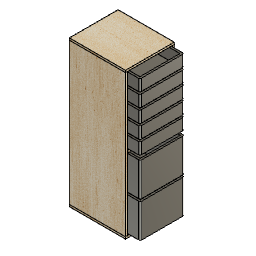
model (Autodesk Fusion 360 design; units mm, degrees)
Autodesk Fusion 360 part; units mm, degrees
note: some values were not read from the file. Chosen so that the rebuilt part matches the saved one: which bodies a step acts on.
sketch "Sketch1" plane through (0, 0, 0) normal (0, 0, 1) x (1, 0, 0) in component "eb432"
  line L0 (15, 0) -> (383, 0)
  line L1 (398, 15) -> (398, 284)
  line L2 (383, 299) -> (15, 299)
  line L3 (0, 284) -> (0, 15)
  arc A0 (15, 299) -> (0, 284) centre (15, 284) ccw
  arc A1 (398, 284) -> (383, 299) centre (383, 284) ccw
  arc A2 (383, 0) -> (398, 15) centre (383, 15) ccw
  arc A3 (0, 15) -> (15, 0) centre (15, 15) ccw
  line L4 (0, 0) -> (18, 18) construction
  line L5 (18, 18) -> (380, 18)
  line L6 (380, 18) -> (380, 281)
  line L7 (380, 281) -> (18, 281)
  line L8 (18, 281) -> (18, 18)
  point P0 (398, 0)
  point P1 (0, 299)
  dimension "d1" = 398
  dimension "d2" = 299
  dimension "d3" = 15
  dimension "d6" = 18
  dimension "d7" = 18
  dimension "d8" = 263
  dimension "d15" = 362
  constraint horizontal L0
  constraint vertical L1
  constraint horizontal L2
  constraint vertical L3
  constraint coincident L4.start origin
  constraint coincident P1 L2
  constraint coincident P1 L3
  constraint tangent L2 A0
  constraint tangent L3 A0
  constraint tangent L1 A1
  constraint tangent L2 A1
  constraint equal A0 A1
  constraint coincident P0 L0
  constraint coincident P0 L1
  constraint tangent L0 A2
  constraint tangent L1 A2
  constraint equal A0 A2
  constraint coincident L4.start L0
  constraint coincident L4.start L3
  constraint tangent L0 A3
  constraint tangent L3 A3
  constraint equal A0 A3
  constraint horizontal L5
  constraint vertical L6
  constraint horizontal L7
  constraint vertical L8
  measures "d1" distance of L4.start P0
  measures "d2" distance of L4.start P1
  measures "d3" radius of A0
  measures "d6" horizontal distance of L4.end L4.start
  measures "d7" vertical distance of L4.end L4.start
  measures "d8" distance of L5.end L6.end
  measures "d15" distance of L6.end L7.end
extrude "Extrude1" add sketch "Sketch1" along normal blind 14 and the other way blind -218 makes body 1 in component "eb432"
extrude "Extrude2" add sketch "Sketch1" along normal blind 14 separate body contours L5 L6 L7 L8 makes body 2 in component "eb432"
sketch "Sketch1 (2)" plane through (0, 0, 0) normal (0, 0, 1) x (1, 0, 0) in component "eb641"
  arc A0 (599, 384) -> (584, 399) centre (584, 384) ccw
  line L0 (0, 384) -> (0, 15)
  line L1 (599, 15) -> (599, 384)
  line L2 (584, 399) -> (15, 399)
  arc A1 (15, 399) -> (0, 384) centre (15, 384) ccw
  arc A2 (0, 15) -> (15, 0) centre (15, 15) ccw
  arc A3 (584, 0) -> (599, 15) centre (584, 15) ccw
  line L3 (581, 381) -> (18, 381)
  line L4 (581, 18) -> (581, 381)
  line L5 (18, 381) -> (18, 18)
  line L6 (18, 18) -> (581, 18)
  line L7 (0, 0) -> (18, 18) construction
  line L8 (15, 0) -> (584, 0)
  point P0 (0, 399)
  point P1 (599, 0)
  dimension "d28" = 599
  dimension "d29" = 399
  dimension "d30" = 15
  dimension "d31" = 18
  dimension "d32" = 18
  dimension "d33" = 363
  dimension "d34" = 563
  constraint horizontal L8
  constraint vertical L1
  constraint horizontal L2
  constraint vertical L0
  constraint coincident L7.start origin
  constraint coincident P0 L2
  constraint coincident P0 L0
  constraint tangent L2 A1
  constraint tangent L0 A1
  constraint tangent A0 L1
  constraint tangent A0 L2
  constraint equal A0 A1
  constraint coincident P1 L8
  constraint coincident P1 L1
  constraint tangent A3 L8
  constraint tangent L1 A3
  constraint equal A1 A3
  constraint coincident L7.start L8
  constraint coincident L7.start L0
  constraint tangent A2 L8
  constraint tangent L0 A2
  constraint equal A1 A2
  constraint horizontal L6
  constraint vertical L4
  constraint horizontal L3
  constraint vertical L5
  measures "d28" distance of P1 L7.start
  measures "d29" distance of P0 L7.start
  measures "d30" radius of A1
  measures "d31" horizontal distance of L7.start L5.end
  measures "d32" vertical distance of L7.start L5.end
  measures "d33" distance of L4.start L3.start
  measures "d34" distance of L3.start L3.end
extrude "Extrude1'" add sketch "Sketch1 (2)" along normal blind 14 separate body contours L3 L4 L5 L6 makes body 3 in component "eb641"
extrude "Extrude2'" add sketch "Sketch1 (2)" along normal blind 14 and the other way blind -118 bodies 3 in component "eb641"
sketch "Sketch1 (3)" plane through (0, 0, 0) normal (0, 0, 1) x (1, 0, 0) in component "eb643"
  line L0 (584, 399) -> (15, 399)
  line L1 (599, 15) -> (599, 384)
  arc A0 (0, 15) -> (15, 0) centre (15, 15) ccw
  line L2 (581, 18) -> (581, 381)
  line L3 (0, 0) -> (18, 18) construction
  line L4 (18, 18) -> (581, 18)
  arc A1 (584, 0) -> (599, 15) centre (584, 15) ccw
  line L5 (15, 0) -> (584, 0)
  arc A2 (599, 384) -> (584, 399) centre (584, 384) ccw
  line L6 (581, 381) -> (18, 381)
  arc A3 (15, 399) -> (0, 384) centre (15, 384) ccw
  line L7 (0, 384) -> (0, 15)
  line L8 (18, 381) -> (18, 18)
  point P0 (0, 399)
  point P1 (599, 0)
  dimension "d41" = 599
  dimension "d42" = 399
  dimension "d43" = 15
  dimension "d44" = 18
  dimension "d45" = 18
  dimension "d46" = 363
  dimension "d47" = 563
  constraint horizontal L5
  constraint vertical L1
  constraint horizontal L0
  constraint vertical L7
  constraint coincident L3.start origin
  constraint coincident P0 L0
  constraint coincident P0 L7
  constraint tangent L0 A3
  constraint tangent A3 L7
  constraint tangent L1 A2
  constraint tangent L0 A2
  constraint equal A2 A3
  constraint coincident P1 L5
  constraint coincident P1 L1
  constraint tangent A1 L5
  constraint tangent L1 A1
  constraint equal A1 A3
  constraint coincident L3.start L5
  constraint coincident L3.start L7
  constraint tangent A0 L5
  constraint tangent A0 L7
  constraint equal A0 A3
  constraint horizontal L4
  constraint vertical L2
  constraint horizontal L6
  constraint vertical L8
  measures "d41" distance of L3.start P1
  measures "d42" distance of P0 L3.start
  measures "d43" radius of A3
  measures "d44" horizontal distance of L3.end L3.start
  measures "d45" vertical distance of L3.end L3.start
  measures "d46" distance of L2.end L2.start
  measures "d47" distance of L2.end L6.end
extrude "Extrude1''" add sketch "Sketch1 (3)" along normal blind 14 separate body contours L2 L4 L6 L8 makes body 4 in component "eb643"
extrude "Extrude2''" add sketch "Sketch1 (3)" along normal blind 14 and the other way blind -318 separate body makes body 5 in component "eb643"
pattern_linear "00000000-0000-0000-0000-000000000000" [suppressed]
pattern_linear "00000000-0000-0000-0000-000000000000'" [suppressed]
sketch "Sketch1 (4)" plane through (0, 0, 0) normal (0, 0, 1) x (1, 0, 0)
  line L0 (0, 0) -> (-21, -3) construction
  line L1 (0, 0) -> (7.0711, 0) construction
  line L2 (-21, -3) -> (487, -3)
  line L3 (487, -3) -> (487, 402)
  line L4 (487, 402) -> (-21, 402)
  line L5 (-21, 402) -> (-21, -3)
  line L6 (-21, 402) -> (487, 402)
  line L7 (487, 402) -> (487, 420)
  line L8 (487, 420) -> (-21, 420)
  line L9 (-21, 420) -> (-21, 402)
  line L10 (-21, -3) -> (487, -3)
  line L11 (487, -3) -> (487, -21)
  line L12 (487, -21) -> (-21, -21)
  line L13 (-21, -21) -> (-21, -3)
  line L14 (-21, -3) -> (-3, -3)
  line L15 (-3, -3) -> (-3, 402)
  line L16 (-3, 402) -> (-21, 402)
  line L17 (-21, 402) -> (-21, -3)
  dimension "d72" = 21
  dimension "d73" = 405
  dimension "d74" = 508
  dimension "d75" = 18
  dimension "d76" = 18
  dimension "d77" = 3
  dimension "d88" = 18
  constraint horizontal L1
  constraint coincident L0.start L1.start
  constraint horizontal L2
  constraint vertical L3
  constraint horizontal L4
  constraint vertical L5
  constraint horizontal L6
  constraint vertical L7
  constraint horizontal L8
  constraint vertical L9
  constraint equal L4 L8
  constraint horizontal L10
  constraint vertical L11
  constraint horizontal L12
  constraint vertical L13
  constraint equal L2 L12
  constraint horizontal L14
  constraint vertical L15
  constraint horizontal L16
  constraint vertical L17
  constraint coincident L6 L15.end
  measures "d72" horizontal distance of L0.start L0.end
  measures "d73" distance of L0.end L4.end
  measures "d74" distance of L0.end L2.end
  measures "d75" distance of L4.end L8.end
  measures "d76" distance of L0.end L12.end
  measures "d77" vertical distance of L0.start L0.end
  measures "d88" distance of L15 L17
extrude "Extrude1'''" add sketch "Sketch1 (4)" against normal blind 18 separate body makes body 6
extrude "Extrude4" add sketch "Sketch1 (4)" along normal blind 100 separate body contours L2 L4 L5 L6 L10 L14 L15 L16 L17 makes body 7
sketch "Sketch2" plane through (0, 0, 642) normal (0, 0, 1) x (-1, 0, 0)
  line L0 (-18, -18) -> (-18, -381)
  line L1 (-18, -381) -> (-581, -381)
  line L2 (-581, -381) -> (-581, -18)
  line L3 (-581, -18) -> (-18, -18)
  line L4 (0, -384) -> (0, -15)
  arc A0 (0, -15) -> (-15, 0) centre (-15, -15) ccw
  line L5 (-15, 0) -> (-584, 0)
  arc A1 (-584, 0) -> (-599, -15) centre (-584, -15) ccw
  line L6 (-599, -15) -> (-599, -384)
  arc A2 (-599, -384) -> (-584, -399) centre (-584, -384) ccw
  line L7 (-584, -399) -> (-15, -399)
  arc A3 (-15, -399) -> (0, -384) centre (-15, -384) ccw
  line L8 (0, 0) -> (21, 3) construction
  line L9 (0, -1.75) -> (0, -22.5) construction
  line L10 (-1.75, 0) -> (-22.5, 0) construction
  line L11 (21, 3) -> (-487, 3)
  line L12 (-487, 3) -> (-487, -402)
  line L13 (-487, -402) -> (21, -402)
  line L14 (21, -402) -> (21, 3)
  dimension "d92" = 21
  dimension "d93" = 3
  dimension "d94" = 405
  dimension "d95" = 508
  constraint coincident L8.start origin
  constraint horizontal L11
  constraint vertical L12
  constraint horizontal L13
  constraint vertical L14
  measures "d92" distance of L8.end L9
  measures "d93" distance of L8.end L10
  measures "d94" distance of L11 L13
  measures "d95" distance of L12 L14
extrude "Extrude5" add sketch "Sketch2" along normal blind 24 and the other way blind -6 separate body contours L0 L1 L3 L4 A0 L5 L7 A3 L12 | L0 L1 L3 L12 | L4 A0 L5 L7 A3 L11 L12 L13 L14 makes body 8
extrude "Extrude6" add sketch "Sketch1 (4)" along normal blind 18 from surface at 1286 separate body makes body 9
extrude "Extrude3" add sketch "Sketch1 (4)" along normal up to near side of body 9 separate body contours L2 L10 L11 L12 L13 L14 | L4 L6 L7 L8 L9 L16 makes body 10 at (148.3333, -3, 428.6667) makes body 11 at (317.6667, 402, 428.6667)
sketch "Sketch3" plane through (0, 0, 1286) normal (0, 0, -1) x (1, 0, 0)
  line L0 (487, 21) -> (-21, 21)
  line L1 (-21, 21) -> (-21, -420)
  line L2 (-21, -420) -> (487, -420)
  line L3 (487, -420) -> (487, 21)
  line L4 (0, 0) -> (-3, 3) construction
  line L5 (-3, 3) -> (-21, 3)
  line L6 (-21, 3) -> (-21, -402)
  line L7 (-21, -402) -> (-3, -402)
  line L8 (-3, -402) -> (-3, 3)
  dimension "d108" = 3
  dimension "d109" = 3
  dimension "d110" = 405
  constraint coincident L4.start origin
  constraint horizontal L5
  constraint vertical L6
  constraint horizontal L7
  constraint vertical L8
  constraint coincident L1 L6.end
  measures "d108" horizontal distance of L4.start L4.end
  measures "d109" vertical distance of L4.start L4.end
  measures "d110" distance of L5 L7
extrude "Extrude7" add sketch "Sketch3" along normal blind 100 separate body contours L1 L5 L6 L7 L8 makes body 12
copy_body "CutPasteBodies1" bodies 12 6 8 7 9 11 10 removing the originals makes body 13 makes body 14 makes body 15 makes body 16 makes body 17 makes body 18 makes body 19 in component "wood"
sketch "Sketch4" plane through (487, 0, 0) normal (1, 0, 0) x (0, 1, 0)
  line L0 (-3, 1286) -> (-21, 1286)
  line L1 (-21, 1286) -> (-21, 0)
  line L2 (-21, 0) -> (-3, 0)
  line L3 (-3, 0) -> (-3, 1286)
  line L4 (-3, 804) -> (5, 804)
  line L5 (5, 804) -> (5, 788)
  line L6 (5, 788) -> (-3, 788)
  line L7 (-3, 788) -> (-3, 804)
  line L8 (0, 0) -> (0, 804) construction
  dimension "d113" = 8
  dimension "d114" = 16
  dimension "d115" = 804
  constraint horizontal L4
  constraint vertical L5
  constraint horizontal L6
  constraint vertical L7
  constraint coincident L3 L4.start
  constraint coincident L8.start origin
  constraint parallel L7 L8
  constraint coincident L4 L8.end
  measures "d113" distance of L4.start L4.end
  measures "d114" distance of L4.start L6.end
  measures "d115" distance of L8.start L8.end
extrude "Extrude8" add sketch "Sketch4" along normal blind -333 and the other way blind 48 separate body contours L3 L4 L5 L6 L7 makes body 20
sketch "Sketch5" plane through (0, 5, 0) normal (0, 1, 0) x (-1, 0, 0)
  line L0 (-439, 804) -> (-439, 788)
  line L1 (-439, 788) -> (-154, 788)
  line L2 (-154, 788) -> (-154, 804)
  line L3 (-154, 804) -> (-439, 804)
  line L4 (-154, 796) -> (-439, 796) construction
  circle A0 centre (-409, 796) radius 1.5
  circle A1 centre (-345, 796) radius 1.5
  circle A2 centre (-249, 796) radius 1.5
  circle A3 centre (-185, 796) radius 1.5
  dimension "d118" = 3
  dimension "d120" = 30
  dimension "d121" = 3
  dimension "d122" = 3
  dimension "d123" = 3
  dimension "d124" = 64
  dimension "d125" = 96
  dimension "d126" = 64
  constraint midpoint L2 L4.start
  constraint midpoint L0 L4.end
  constraint coincident L4 A0.centre
  constraint coincident L4 A1.centre
  constraint coincident L4 A2.centre
  constraint coincident L4 A3.centre
  measures "d118" diameter of A0
  measures "d120" distance of L0 A0.centre
  measures "d121" diameter of A1
  measures "d122" diameter of A2
  measures "d123" diameter of A3
  measures "d124" distance of A0.centre A1.centre
  measures "d125" distance of A1.centre A2.centre
  measures "d126" distance of A2.centre A3.centre
extrude "Extrude9" cut sketch "Sketch5" against normal blind 8 contours A0 | A1 | A2 | A3 bodies 20
chamfer "Chamfer1" distance 1.5 angle 45 4 edges at (410.3985, 5, 796.5424) (346.3985, 5, 796.5424) (250.3985, 5, 796.5424) (186.3985, 5, 796.5424) on bodies 20
fillet "Fillet1" radius 2 8 edges at (439, 5, 796) (439, 1, 804) (296.5, 5, 804) (296.5, 5, 788) (154, 5, 796) (154, 1, 788) (154, 1, 804) (439, 1, 788) on bodies 20
pattern_linear "R-Pattern1" count 4 spacing 124 along (0, 0, 1) of bodies 20 makes body 21 at (165.1667, -3, 920) makes body 22 at (165.1667, -3, 1044) makes body 23 at (165.1667, -3, 1168)
pattern_linear "R-Pattern2" count 2 spacing 466 along (0, 0, -1) of bodies 20 makes body 24
ref_plane "WorkPlane1" through (233, 199.5, 643) normal (0, 1, 0) x (-1, 0, 0)
mirror "Mirror1" about plane through (233, 199.5, 643) normal (0, 1, 0) of bodies 23 22 21 20 24 makes body 25 at (165.1667, 402, 796) makes body 26 at (165.1667, 402, 920) makes body 27 at (165.1667, 402, 1044) makes body 28 at (165.1667, 402, 1168) makes body 29 at (165.1667, 402, 330)
copy_body "CutPasteBodies1'" bodies 20 22 25 26 27 28 29 21 24 23 removing the originals makes body 30 makes body 31 makes body 32 makes body 33 makes body 34 makes body 35 makes body 36 makes body 37 makes body 38 makes body 39 in component "rails"
component "wood" placed x (1, 0, 0) y (0, 1, 0) z (0, 0, 1) at (0, 0, 0)
component "rails" placed x (1, 0, 0) y (0, 1, 0) z (0, 0, 1) at (0, 0, 0)
component "boxes" placed x (1, 0, 0) y (0, 1, 0) z (0, 0, 1) at (0, 0, 0)
component "eb641" placed x (1, 0, 0) y (0, 1, 0) z (0, 0, 1) at (-3, 0, 1162) in component "eb641s"
component "eb641" placed x (1, 0, 0) y (0, 1, 0) z (0, 0, 1) at (-3, 0, 1038) in component "eb641s"
component "eb641" placed x (1, 0, 0) y (0, 1, 0) z (0, 0, 1) at (-3, 0, 914) in component "eb641s"
component "eb641" placed x (1, 0, 0) y (0, 1, 0) z (0, 0, 1) at (-3, 0, 790) in component "eb641s"
component "eb641" placed x (1, 0, 0) y (0, 1, 0) z (0, 0, 1) at (-3, 0, 666) in component "eb641s"
component "eb643" placed x (1, 0, 0) y (0, 1, 0) z (0, 0, 1) at (0, 0, 324) in component "eb643s"
component "eb643" placed x (1, 0, 0) y (0, 1, 0) z (0, 0, 1) at (0, 0, 0) in component "eb643s"
component "eb643s" placed x (1, 0, 0) y (0, 1, 0) z (0, 0, 1) at (0, 0, 0) in component "boxes"
component "eb432" placed x (1, 0, 0) y (0, 1, 0) z (0, 0, 1) at (0, 0, 0) in component "boxes"
component "eb641s" placed x (1, 0, 0) y (0, 1, 0) z (0, 0, 1) at (0, 0, 0) in component "boxes"
equation "d1 = eb432_width"
equation "d2 = eb432_depth"
equation "d3 = eb_radius"
equation "d6 = eb_overhang"
equation "d7 = eb_overhang"
equation "d8 = eb432_depth - ( eb_overhang * 2 )"
equation "eb_overhang = 18 mm"
equation "eb_overlap = 14 mm"
equation "eb432_width = 398 mm"
equation "eb432_height = 204 mm"
equation "eb432_depth = 299 mm"
equation "eb_radius = 15 mm"
equation "d15 = eb432_width - ( 2 * eb_overhang )"
equation "d16 = eb_overlap"
equation "d18 = -eb432_height - eb_overlap"
equation "d20 = eb_overlap"
equation "eb64_width = 599 mm"
equation "eb641_height = 104 mm"
equation "eb64_depth = 399 mm"
equation "eb643_height = 304 mm"
equation "d28 = eb64_width"
equation "d29 = eb64_depth"
equation "d30 = eb_radius"
equation "d31 = eb_overhang"
equation "d32 = eb_overhang"
equation "d33 = eb64_depth - ( eb_overhang * 2 )"
equation "d34 = eb64_width - ( 2 * eb_overhang )"
equation "d35 = eb_overlap"
equation "d37 = eb_overlap"
equation "d39 = -eb641_height - eb_overlap"
equation "d41 = eb64_width"
equation "d42 = eb64_depth"
equation "d43 = eb_radius"
equation "d44 = eb_overhang"
equation "d45 = eb_overhang"
equation "d46 = eb64_depth - ( eb_overhang * 2 )"
equation "d47 = eb64_width - ( 2 * eb_overhang )"
equation "d48 = eb_overlap"
equation "d50 = eb_overlap"
equation "d52 = -eb643_height - eb_overlap"
equation "shelf_vmargin = 6 mm"
equation "d57 = eb643_height + eb_overlap + shelf_vmargin"
equation "panel_thickness = 18 mm"
equation "shelf_hmargin = 3 mm"
equation "d63 = eb641_height + eb_overlap + shelf_vmargin"
equation "rail_height = 16 mm"
equation "panel_width = 20 in"
equation "d72 = panel_thickness + shelf_hmargin"
equation "d73 = eb64_depth + ( 2 * shelf_hmargin )"
equation "d74 = panel_width"
equation "d75 = panel_thickness"
equation "d76 = panel_thickness"
equation "rail_thickness = 8 mm"
equation "rail_length = 285 mm"
equation "d80 = -panel_thickness"
equation "d88 = panel_thickness"
equation "kick_height = 100 mm"
equation "d90 = kick_height"
equation "d92 = shelf_hmargin + panel_thickness"
equation "d93 = shelf_hmargin"
equation "d94 = eb64_depth + ( 2 * shelf_hmargin )"
equation "d95 = panel_width"
equation "d96 = panel_thickness + shelf_vmargin"
equation "d98 = -shelf_vmargin"
equation "d102 = eb_overlap"
equation "d103 = -panel_thickness"
equation "d104 = shelf_vmargin"
equation "d105 = panel_thickness"
equation "d108 = shelf_hmargin"
equation "d109 = shelf_hmargin"
equation "d110 = eb64_depth + ( 2 * shelf_hmargin )"
equation "d111 = kick_height"
equation "d113 = rail_thickness"
equation "d114 = rail_height"
equation "d115 = 2 * eb643_height + 3 * shelf_vmargin + panel_thickness + 4 * eb_overlap + eb641_height"
equation "d116 = -rail_length - rail_front_inset"
equation "d118 = rail_hole_diameter"
equation "rail_hole_diameter = 3 mm"
equation "d121 = rail_hole_diameter"
equation "d122 = rail_hole_diameter"
equation "d123 = rail_hole_diameter"
equation "d127 = -rail_thickness"
equation "d129 = rail_hole_diameter / 2"
equation "d131 = rail_thickness / 4"
equation "rail_front_inset = ( eb64_width - rail_length ) / 2 - ( eb64_width - panel_width ) - panel_thickness"
equation "d133 = rail_front_inset"
equation "d137 = eb641_height + eb_overlap + shelf_vmargin"
equation "d141 = -( eb641_height + eb643_height + panel_thickness + 2 * eb_overlap + 2 * shelf_vmargin )"
